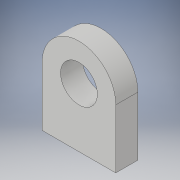
# Autodesk Inventor part: SUJECION_BALSA_UNDIMOTRIZ
Saved by Autodesk Inventor 2019.4 (Build 234330000, 330)
## iProperties
Created: 2020-08-20
Part Number: SUJECION_BALSA_UNDIMOTRIZ
Material: Generic
Document SubType Name: Modeling
Designer: crist
Density: 1 g/cm^3
Appearance: Default
Author: crist
Autodesk Inventor part; units mm, degrees
ref_plane "YZ Plane" through (0, 0, 0) normal (1, 0, 0) x (0, 1, 0)
ref_plane "XZ Plane" through (0, 0, 0) normal (0, 1, 0) x (-1, 0, 0)
ref_plane "XY Plane" through (0, 0, 0) normal (0, 0, 1) x (1, 0, 0)
sketch "Boceto2" plane through (0, 0, 0) normal (0, 0, 1) x (1, 0, 0)
  circle A0 centre (0, 0) radius 250
  circle A1 centre (0, 0) radius 125
  line L0 (250, 0) -> (250, -400)
  line L1 (250, -400) -> (-250, -400)
  line L2 (-250, -400) -> (-250, 0)
  dimension "d7" = 500
  dimension "d8" = 250
  dimension "d9" = 400
  dimension "d10" = 500
  constraints: 6 end point, 2 centre point, 2 coincident, 2 point on circle, 2 tangent, 1 perpendicular, 1 vertical
  measures "d7" diameter of A0
  measures "d8" diameter of A1
  measures "d9" distance of L0.start L0.end
  measures "d10" distance of L0.end L1.end
extrude "Extrusión2" add sketch "Boceto2" along normal blind 150
